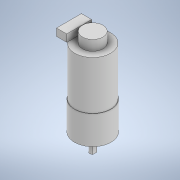
# Autodesk Inventor part: 7_Motore
Saved by Autodesk Inventor 2020.2 (Build 242310000, 310)
## iProperties
Created: 2019-10-14
Part Number: 7_Motore
Material: Generico
Document SubType Name: Modeling
Designer: socci
Density: 1 g/cm^3
Appearance: Default
Author: socci
Autodesk Inventor part; units mm, degrees
ref_plane "YZ Plane" through (0, 0, 0) normal (1, 0, 0) x (0, 1, 0)
ref_plane "XZ Plane" through (0, 0, 0) normal (0, 1, 0) x (-1, 0, 0)
ref_plane "XY Plane" through (0, 0, 0) normal (0, 0, 1) x (1, 0, 0)
sketch "Schizzo1" plane through (0, 0, 0) normal (0, 1, 0) x (-1, 0, 0)
  circle A0 centre (0, 0) radius 12.2
  dimension "d0" = 24.4
  constraints: 1 centre point, 1 coincident
  measures "d0" diameter of A0
extrude "Estrusione1" add sketch "Schizzo1" along normal blind 31
sketch "Schizzo2" plane through (0, 0, 0) normal (0, -1, 0) x (1, 0, 0)
  circle A0 centre (0, 0) radius 12.5
  dimension "d3" = 25
  constraints: 1 centre point, 1 coincident
  measures "d3" diameter of A0
extrude "Estrusione2" add sketch "Schizzo2" along normal blind 19.5
sketch "Schizzo3" plane through (0, -19.5, 0) normal (0, -1, 0) x (1, 0, 0)
  circle A0 centre (0, 0) radius 12.2 projected
  circle A1 centre (0, 0) radius 3.5
  dimension "d6" = 7
  constraints: 1 centre point, 1 coincident
  measures "d6" diameter of A1
extrude "Estrusione3" add sketch "Schizzo3" along normal blind 2.5 contours A1
sketch "Schizzo4" plane through (0, -22, 0) normal (0, -1, 0) x (1, 0, 0)
  circle A0 centre (0, 0) radius 2
  dimension "d9" = 4
  constraints: 1 centre point, 1 coincident
  measures "d9" diameter of A0
extrude "Estrusione4" add sketch "Schizzo4" along normal blind 9.5
sketch "Schizzo5" plane through (0, -31.5, 0) normal (0, -1, 0) x (1, 0, 0)
  circle A0 centre (0, 0) radius 2 projected
  line L0 (-2, 0) -> (1.5, 0)
  line L1 (1.5, 0) -> (1.5, -1.3229)
  line L2 (1.5, 0) -> (1.5, 1.3229)
  dimension "d12" = 3.5
  constraints: 6 end point, 3 point on circle, 1 horizontal, 1 perpendicular, 1 vertical
  measures "d12" distance of L0.start L0.end
extrude "Estrusione5" cut sketch "Schizzo5" against normal blind 8 contours A0 L1 L2
sketch "Schizzo6" plane through (0, -19.5, 0) normal (0, -1, 0) x (1, 0, 0)
  line L0 (0, 0) -> (8.5, 0)
  circle A0 centre (8.5, 0) radius 1.5
  line L1 (8.5, 0) -> (-8.5, 0)
  line L2 (8.5, 0) -> (25.5, 0) construction
  circle A1 centre (-8.5, 0) radius 1.5
  dimension "d15" = 8.5
  dimension "d16" = 3
  dimension "d17" = 17
  dimension "d18" = 180
  dimension "d19" = 3
  constraints: 6 end point, 3 horizontal, 2 centre point, 2 coincident, 1 collinear
  measures "d15" distance of L0.start L0.end
  measures "d16" diameter of A0
  measures "d17" distance of L1.start L1.end
  measures "d18" angle of L1 L2
  measures "d19" diameter of A1
hole "Foro1" at (8.5, -19.5, 0) at (-8.5, -19.5, 0) direction (0, 1, 0) diameter 2.459 depth 8.8 tip angle 118 thread size "M3x0.5" class "6H" standard "ANSI Metric M Profile"
sketch "Schizzo7" plane through (0, 31, 0) normal (0, 1, 0) x (1, 0, 0)
  point P0 (0, 0)
sketch "Schizzo8" plane through (0, 31, 0) normal (0, 1, 0) x (1, 0, 0)
  circle A0 centre (0, 0) radius 7
  dimension "d30" = 14
  constraints: 1 centre point
  measures "d30" diameter of A0
extrude "Estrusione6" add sketch "Schizzo8" along normal blind 9 from surface at 0
sketch "Schizzo9" plane through (0, 31, 0) normal (0, 1, 0) x (1, 0, 0)
  circle A0 centre (0, 0) radius 12.2
  dimension "d31" = 24.4
  constraints: 1 centre point, 1 coincident
  measures "d31" diameter of A0
extrude "Estrusione7" add sketch "Schizzo9" along normal blind 2
sketch "Schizzo10" plane through (0, 33, 0) normal (0, 1, 0) x (1, 0, 0)
  circle A0 centre (0, 0) radius 12.2 projected
  line L0 (-12.2, 0) -> (-9.2, 0)
  line L1 (-9.2, 8.5) -> (-16.2, 8.5)
  line L2 (-16.2, 8.5) -> (-16.2, -8.5)
  line L3 (-16.2, -8.5) -> (-9.2, -8.5)
  line L4 (-9.2, -8.5) -> (-9.2, 8.5)
  dimension "d34" = 3
  dimension "d35" = 17
  dimension "d36" = 7
  constraints: 10 end point, 2 horizontal, 2 parallel, 1 horizontal alignment, 1 midpoint, 1 perpendicular, 1 other
  measures "d34" distance of L0.end L0.start
  measures "d35" distance of L3.end L1.start
  measures "d36" distance of L1.end L1.start
extrude "Estrusione8" add sketch "Schizzo10" along normal blind 5 contours L4 L0 A0 | A0 L4 L3 L2 L1 | A0 L0 L4
